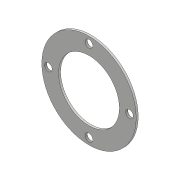
# Autodesk Inventor part: BiggerFanFlange
Saved by Autodesk Inventor 2017 (Build 210142000, 142)
## iProperties
Created: 2017-05-22
Part Number: BiggerFanFlange
Material: Generic
Document SubType Name: Modeling
Designer: krosie
Density: 1 g/cm^3
Appearance: Default
Author: krosie
Autodesk Inventor part; units mm, degrees
ref_plane "YZ Plane" through (0, 0, 0) normal (1, 0, 0) x (0, 1, 0)
ref_plane "XZ Plane" through (0, 0, 0) normal (0, 1, 0) x (-1, 0, 0)
ref_plane "XY Plane" through (0, 0, 0) normal (0, 0, 1) x (1, 0, 0)
sketch "Sketch1" plane through (0, 0, 0) normal (0, 1, 0) x (-1, 0, 0)
  circle A0 centre (0, 0) radius 52.7 construction
  circle A1 centre (0, 0) radius 55 construction
  circle A2 centre (0, 0) radius 57 construction
  circle A3 centre (0, 0) radius 30
  circle A4 centre (0, 0) radius 46.5
  circle A5 centre (0, 0) radius 40 construction
  circle A6 centre (40, 0) radius 3.75
  circle A7 centre (0, -40) radius 3.75
  circle A8 centre (-40, 0) radius 3.75
  circle A9 centre (0, 40) radius 3.75
  dimension "d0" = 105.4
  dimension "d1" = 110
  dimension "d2" = 114
  dimension "d3" = 60
  dimension "d4" = 93
  dimension "d5" = 80
  dimension "d6" = 7.5
  dimension "d7" = 7.5
  dimension "d8" = 7.5
  dimension "d9" = 7.5
  constraints: 10 centre point, 10 coincident, 4 point on circle
  measures "d0" diameter of A0
  measures "d1" diameter of A1
  measures "d2" diameter of A2
  measures "d3" diameter of A3
  measures "d4" diameter of A4
  measures "d5" diameter of A5
  measures "d6" diameter of A6
  measures "d7" diameter of A7
  measures "d8" diameter of A8
  measures "d9" diameter of A9
extrude "Extrusion1" add sketch "Sketch1" along normal blind 2
body "Solid1"
